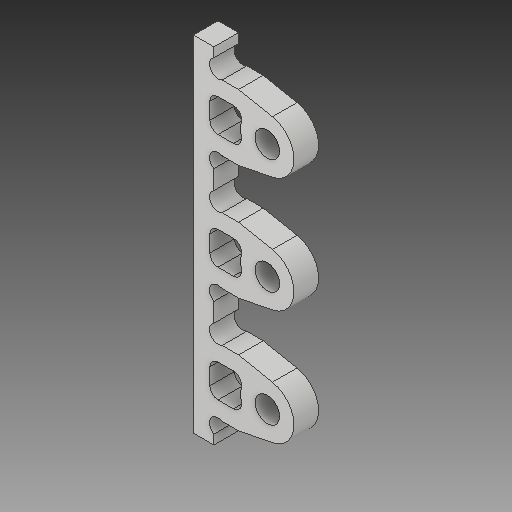
# Autodesk Inventor part: アームユニット底板締結パーツ3t用(2)
Saved by Autodesk Inventor 2020 (Build 240168000, 168)
## iProperties
Created: 2018-11-28
Part Number: アームユニット底板締結パーツ3t用(2)
Material: アルミニウム 2014-T4
Document SubType Name: Modeling
Designer: 雪村
Density: 2.8 g/cm^3
Appearance: サテン
Mass: 1.96677 g
Surface Area: 10.9285 cm^2
Volume: 0.702418 cm^3
Description: アルミ2000 3t
Author: 雪村
Autodesk Inventor part; units mm, degrees
ref_plane "YZ Plane" through (0, 0, 0) normal (1, 0, 0) x (0, 1, 0)
ref_plane "XZ Plane" through (0, 0, 0) normal (0, 1, 0) x (-1, 0, 0)
ref_plane "XY Plane" through (0, 0, 0) normal (0, 0, 1) x (1, 0, 0)
sketch "スケッチ1" plane through (0, 0, 0) normal (0, 0, 1) x (1, 0, 0)
  line L0 (-7, -29) -> (-7, -27)
  arc A0 (-6, -26) -> (-7, -27) centre (-6, -27) ccw
  line L1 (-6, -26) -> (-4.1307, -26)
  arc A1 (-3.1588, -27.2353) -> (-4.1307, -26) centre (-4.1307, -27) ccw
  arc A2 (-3.1588, -27.2353) -> (-3.1588, -28.7647) centre (0, -28) ccw
  arc A3 (-4.1307, -30) -> (-3.1588, -28.7647) centre (-4.1307, -29) ccw
  line L2 (-4.1307, -30) -> (-6, -30)
  arc A4 (-7, -29) -> (-6, -30) centre (-6, -29) ccw
  arc A5 (-6.5, -22.1534) -> (-5.5, -24) centre (-6, -23.0767) ccw
  line L3 (-6.5, -21) -> (-6.5, -22.1534)
  line L4 (-9, -21) -> (-6.5, -21)
  line L5 (-9, -35) -> (-9, -21)
  line L6 (-6.5, -35) -> (-9, -35)
  line L7 (-6.5, -33.8466) -> (-6.5, -35)
  arc A6 (-5.5, -32) -> (-6.5, -33.8466) centre (-6, -32.9233) ccw
  line L8 (-3.5, -32) -> (-5.5, -32)
  line L9 (0.6267, -31.189) -> (-3.5, -32)
  arc A7 (0.6267, -31.189) -> (0.6267, -24.811) centre (0, -28) ccw
  line L10 (-3.5, -24) -> (0.6267, -24.811)
  line L11 (-5.5, -24) -> (-3.5, -24)
  circle A8 centre (0, -28) radius 1.25
  line L12 (-7, -15) -> (-7, -13)
  arc A9 (-6, -12) -> (-7, -13) centre (-6, -13) ccw
  line L13 (-6, -12) -> (-4.1307, -12)
  arc A10 (-3.1588, -13.2353) -> (-4.1307, -12) centre (-4.1307, -13) ccw
  arc A11 (-3.1588, -13.2353) -> (-3.1588, -14.7647) centre (0, -14) ccw
  arc A12 (-4.1307, -16) -> (-3.1588, -14.7647) centre (-4.1307, -15) ccw
  line L14 (-4.1307, -16) -> (-6, -16)
  arc A13 (-7, -15) -> (-6, -16) centre (-6, -15) ccw
  arc A14 (-6.5, -8.1534) -> (-5.5, -10) centre (-6, -9.0767) ccw
  line L15 (-6.5, -7) -> (-6.5, -8.1534)
  line L16 (-9, -7) -> (-6.5, -7)
  line L17 (-9, -21) -> (-9, -7)
  line L18 (-6.5, -21) -> (-9, -21)
  line L19 (-6.5, -19.8466) -> (-6.5, -21)
  arc A15 (-5.5, -18) -> (-6.5, -19.8466) centre (-6, -18.9233) ccw
  line L20 (-3.5, -18) -> (-5.5, -18)
  line L21 (0.6267, -17.189) -> (-3.5, -18)
  arc A16 (0.6267, -17.189) -> (0.6267, -10.811) centre (0, -14) ccw
  line L22 (-3.5, -10) -> (0.6267, -10.811)
  line L23 (-5.5, -10) -> (-3.5, -10)
  circle A17 centre (0, -14) radius 1.25
  line L24 (-7, -1) -> (-7, 1)
  arc A18 (-6, 2) -> (-7, 1) centre (-6, 1) ccw
  line L25 (-6, 2) -> (-4.1307, 2)
  arc A19 (-3.1588, 0.7647) -> (-4.1307, 2) centre (-4.1307, 1) ccw
  arc A20 (-3.1588, 0.7647) -> (-3.1588, -0.7647) centre (0, 0) ccw
  arc A21 (-4.1307, -2) -> (-3.1588, -0.7647) centre (-4.1307, -1) ccw
  line L26 (-4.1307, -2) -> (-6, -2)
  arc A22 (-7, -1) -> (-6, -2) centre (-6, -1) ccw
  arc A23 (-6.5, 5.8466) -> (-5.5, 4) centre (-6, 4.9233) ccw
  line L27 (-6.5, 7) -> (-6.5, 5.8466)
  line L28 (-9, 7) -> (-6.5, 7)
  line L29 (-9, -7) -> (-9, 7)
  line L30 (-6.5, -7) -> (-9, -7)
  line L31 (-6.5, -5.8466) -> (-6.5, -7)
  arc A24 (-5.5, -4) -> (-6.5, -5.8466) centre (-6, -4.9233) ccw
  line L32 (-3.5, -4) -> (-5.5, -4)
  line L33 (0.6267, -3.189) -> (-3.5, -4)
  arc A25 (0.6267, -3.189) -> (0.6267, 3.189) centre (0, 0) ccw
  line L34 (-3.5, 4) -> (0.6267, 3.189)
  line L35 (-5.5, 4) -> (-3.5, 4)
  circle A26 centre (0, 0) radius 1.25
  constraints: 72 end point, 48 point on circle, 27 centre point, 17 horizontal, 12 vertical, 117 other
extrude "押し出し1" add sketch "スケッチ1" along normal blind 3
sketch "スケッチ2" plane through (0, 0, 3) normal (0, 0, 1) x (1, 0, 0)
  arc A0 (-6, 2) -> (-7, 1) centre (-6, 1) ccw projected
  line L0 (-6, 2) -> (-4.1307, 2) projected
  arc A1 (-3.1588, 0.7647) -> (-4.1307, 2) centre (-4.1307, 1) ccw projected
  arc A2 (-3.1588, 0.7647) -> (-3.1588, -0.7647) centre (0, 0) ccw projected
  arc A3 (-4.1307, -2) -> (-3.1588, -0.7647) centre (-4.1307, -1) ccw projected
  line L1 (-4.1307, -2) -> (-6, -2) projected
  arc A4 (-7, -1) -> (-6, -2) centre (-6, -1) ccw projected
  line L2 (-7, -1) -> (-7, 1) projected
  circle A5 centre (0, 0) radius 1.25 projected
  arc A6 (-4.1307, -30) -> (-3.1588, -28.7647) centre (-4.1307, -29) ccw projected
  line L3 (-4.1307, -30) -> (-6, -30) projected
  arc A7 (-7, -29) -> (-6, -30) centre (-6, -29) ccw projected
  line L4 (-7, -29) -> (-7, -27) projected
  arc A8 (-6, -26) -> (-7, -27) centre (-6, -27) ccw projected
  line L5 (-6, -26) -> (-4.1307, -26) projected
  arc A9 (-3.1588, -27.2353) -> (-4.1307, -26) centre (-4.1307, -27) ccw projected
  arc A10 (-3.1588, -27.2353) -> (-3.1588, -28.7647) centre (0, -28) ccw projected
  circle A11 centre (0, -28) radius 1.25 projected
  arc A12 (-6, -12) -> (-7, -13) centre (-6, -13) ccw projected
  line L6 (-6, -12) -> (-4.1307, -12) projected
  arc A13 (-3.1588, -13.2353) -> (-4.1307, -12) centre (-4.1307, -13) ccw projected
  arc A14 (-3.1588, -13.2353) -> (-3.1588, -14.7647) centre (0, -14) ccw projected
  arc A15 (-4.1307, -16) -> (-3.1588, -14.7647) centre (-4.1307, -15) ccw projected
  line L7 (-4.1307, -16) -> (-6, -16) projected
  arc A16 (-7, -15) -> (-6, -16) centre (-6, -15) ccw projected
  line L8 (-7, -15) -> (-7, -13) projected
  circle A17 centre (0, -14) radius 1.25 projected
  arc A18 (-6.5, -8.1534) -> (-5.5, -10) centre (-6, -9.0767) ccw projected
  line L9 (-6.5, -8.1534) -> (-6.5, -5.8466) projected
  arc A19 (-5.5, -4) -> (-6.5, -5.8466) centre (-6, -4.9233) ccw projected
  line L10 (-5.5, -4) -> (-3.5, -4) projected
  line L11 (-3.5, -4) -> (0.6267, -3.189) projected
  arc A20 (0.6267, -3.189) -> (0.6267, 3.189) centre (0, 0) ccw projected
  line L12 (0.6267, 3.189) -> (-3.5, 4) projected
  line L13 (-3.5, 4) -> (-5.5, 4) projected
  arc A21 (-6.5, 5.8466) -> (-5.5, 4) centre (-6, 4.9233) ccw projected
  line L14 (-6.5, 5.8466) -> (-6.5, 7) projected
  line L15 (-6.5, 7) -> (-9, 7) projected
  line L16 (-9, 7) -> (-9, -35) projected
  line L17 (-9, -35) -> (-6.5, -35) projected
  line L18 (-6.5, -35) -> (-6.5, -33.8466) projected
  arc A22 (-5.5, -32) -> (-6.5, -33.8466) centre (-6, -32.9233) ccw projected
  line L19 (-5.5, -32) -> (-3.5, -32) projected
  line L20 (-3.5, -32) -> (0.6267, -31.189) projected
  arc A23 (0.6267, -31.189) -> (0.6267, -24.811) centre (0, -28) ccw projected
  line L21 (0.6267, -24.811) -> (-3.5, -24) projected
  line L22 (-3.5, -24) -> (-5.5, -24) projected
  arc A24 (-6.5, -22.1534) -> (-5.5, -24) centre (-6, -23.0767) ccw projected
  line L23 (-6.5, -22.1534) -> (-6.5, -19.8466) projected
  arc A25 (-5.5, -18) -> (-6.5, -19.8466) centre (-6, -18.9233) ccw projected
  line L24 (-5.5, -18) -> (-3.5, -18) projected
  line L25 (-3.5, -18) -> (0.6267, -17.189) projected
  arc A26 (0.6267, -17.189) -> (0.6267, -10.811) centre (0, -14) ccw projected
  line L26 (0.6267, -10.811) -> (-3.5, -10) projected
  line L27 (-3.5, -10) -> (-5.5, -10) projected
  circle A27 centre (0, 0) radius 1.5
  circle A28 centre (0, -14) radius 1.5
  circle A29 centre (0, -28) radius 1.5
  dimension "d27" = 3
  dimension "d28" = 3
  dimension "d29" = 3
  constraints: 3 centre point, 3 coincident
  measures "d27" diameter of A27
  measures "d28" diameter of A28
  measures "d29" diameter of A29
extrude "押し出し2" cut sketch "スケッチ2" against normal blind 3 contours A27 | A28 | A29
